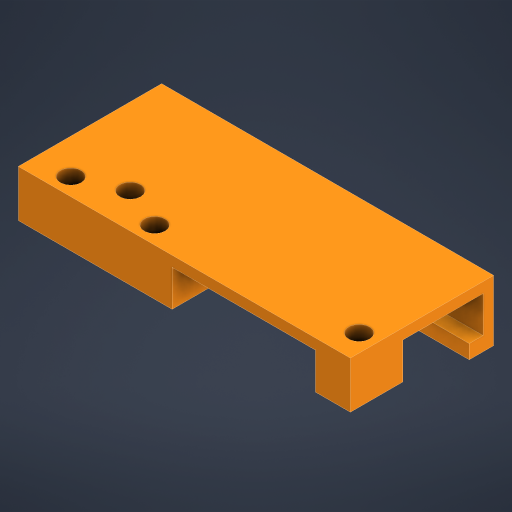
# Autodesk Inventor part: Receptacle_V2
Saved by Autodesk Inventor 2024.1 (Build 281209000, 209)
## iProperties
Created: 2023-05-18
Part Number: Receptacle_V2
Material: PC/ABS Plastic
Document SubType Name: Modeling
Designer: jaege
Density: 1.1 g/cm^3
Appearance: Orange
Mass: 31.7648 g
Surface Area: 177.843 cm^2
Volume: 29.9668 cm^3
Author: jaege
## iProperties of the stored document Receptacle_V2_3DPrint.ipt
Created: 2023-05-19
Part Number: Receptacle_V2_3DPrint
Material: Generic
Document SubType Name: Modeling
Designer: jaege
Density: 1 g/cm^3
Appearance: Default
Author: jaege
Autodesk Inventor part; units mm, degrees
ref_plane "YZ Plane" through (0, 0, 0) normal (1, 0, 0) x (0, 1, 0)
ref_plane "XZ Plane" through (0, 0, 0) normal (0, 1, 0) x (-1, 0, 0)
ref_plane "XY Plane" through (0, 0, 0) normal (0, 0, 1) x (1, 0, 0)
sketch "Sketch1" plane through (0, 0, 0) normal (1, 0, 0) x (0, 1, 0)
  line L0 (-4.7, -13.5) -> (-8.7, -13.5)
  line L1 (-8.7, -13.5) -> (-8.7, -20.5)
  line L2 (-8.7, -20.5) -> (8.7, -20.5)
  line L3 (8.7, -20.5) -> (8.7, 20.5)
  line L4 (8.7, 20.5) -> (-4.7, 20.5)
  line L5 (-4.7, 20.5) -> (-4.7, 5.5)
  line L6 (-4.7, 5.5) -> (5.7, 5.5)
  line L7 (5.7, 5.5) -> (5.7, -17.5)
  line L8 (5.7, -17.5) -> (-4.7, -17.5)
  line L9 (-4.7, -17.5) -> (-4.7, -13.5)
  line L10 (8.7, 20.5) -> (-8.7, -20.5) construction
  point P0 (0, 0)
  point P1 (0, 0)
  dimension "d0" = 4
  dimension "d1" = 4
  dimension "d2" = 10.4
  dimension "d3" = 3
  dimension "d4" = 3
  dimension "d5" = 23
  dimension "d6" = 10.4
  dimension "d7" = 15
  constraints: 22 end point, 8 perpendicular, 1 coincident, 1 horizontal, 1 midpoint, 1 vertical
  measures "d0" distance between parallel lines of L1 L9
  measures "d1" distance between parallel lines of L8 L0
  measures "d2" distance of L7.end L8.end
  measures "d3" distance between parallel lines of L2 L8
  measures "d4" distance between parallel lines of L3 L7
  measures "d5" distance between parallel lines of L6 L8
  measures "d6" distance of L5.end L6.end
  measures "d7" distance of L4.end L5.end
extrude "Outline" add sketch "Sketch1" along normal mid plane 95
sketch "Sketch3" plane through (-47.5, -4.7, 20.5) normal (0, 0, 1) x (1, 0, 0)
  line L0 (0, 0) -> (95, 0) projected
  line L1 (85, 0) -> (44, 0)
  line L2 (44, 0) -> (44, 10.4)
  line L3 (44, 10.4) -> (85, 10.4)
  line L4 (85, 10.4) -> (85, 0)
  line L5 (95, 13.4) -> (95, 0) projected
  line L6 (0, 0) -> (0, 13.4) projected
  line L7 (0, 10.4) -> (95, 10.4) projected
  line L8 (95, 0) -> (95, 10.4) projected
  line L9 (0, 0) -> (95, 0) projected
  line L10 (0, 10.4) -> (0, 0) projected
  point P0 (47.5, 4.7)
  point P1 (44, 0)
  dimension "d22" = 44
  dimension "d26" = 10
  constraints: 8 end point, 2 parallel, 1 collinear, 1 horizontal, 1 perpendicular, 1 point on line
  measures "d22" distance between parallel lines of L6 L2
  measures "d26" distance between parallel lines of L5 L4
extrude "DriverCutout" cut sketch "Sketch3" against normal up to next contours L2 L3 L4 L0
sketch "Sketch2" plane through (-47.5, 8.7, 20.5) normal (0, 1, 0) x (1, 0, 0)
  line L0 (0, 15) -> (44, 15) projected
  line L1 (95, 0) -> (95, 15) projected
  line L2 (0, 0) -> (44, 0) projected
  line L3 (0, 15) -> (0, 0) projected
  line L4 (85, 0) -> (85, 15) projected
  line L5 (85, 15) -> (95, 15) projected
  line L6 (85, 0) -> (95, 0) projected
  line L7 (44, 15) -> (44, 0) projected
  line L8 (10, 5) -> (22, 10) construction
  line L9 (22, 10) -> (34, 5) construction
  line L10 (85, 0) -> (85, 15) construction
  line L11 (34, 5) -> (44, 5) construction
  line L12 (44, 0) -> (44, 15) construction
  line L13 (10, 5) -> (0, 5) construction
  line L14 (85, 15) -> (95, 0) construction
  point P0 (47.5, 20.5)
  point P1 (90, 7.5)
  dimension "d27" = 5
  dimension "d28" = 5
  dimension "d29" = 10
  constraints: 10 end point, 3 point on line, 2 equal length, 1 horizontal alignment, 1 midpoint
  measures "d27" distance between parallel lines of L2 L11
  measures "d28" distance from line of L0 L8.end
  measures "d29" distance from line of L9.end L12
hole "ScrewHoles" at (-37.5, 8.7, 15.5) at (-25.5, 8.7, 10.5) at (-13.5, 8.7, 15.5) at (42.5, 8.7, 13) direction (0, -1, 0) diameter 3.1 depth 13.4 counterbore diameter 6 counterbore depth 9.4
body "Solid1"
